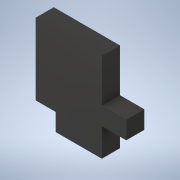
# Autodesk Inventor part: Remote Batery Spacer
Saved by Autodesk Inventor 2020 (Build 240168000, 168)
## iProperties
Created: 2019-06-21
Part Number: Remote Batery Spacer
Material: Generic
Document SubType Name: Modeling
Designer: LSabe
Density: 1 g/cm^3
Appearance: Default
Author: LSabe
Autodesk Inventor part; units mm, degrees
ref_plane "YZ Plane" through (0, 0, 0) normal (1, 0, 0) x (0, 1, 0)
ref_plane "XZ Plane" through (0, 0, 0) normal (0, 1, 0) x (-1, 0, 0)
sketch "Sketch1" plane through (0, 0, 0) normal (0, 0, 1) x (1, 0, 0)
  line L0 (11.176, -4.445) -> (1.27, -4.445)
  line L1 (-5.4348, 0) -> (-5.4348, -19.4068)
  line L2 (12.446, 0) -> (12.446, -11.684)
  line L3 (19.05, -11.684) -> (19.05, -16.51)
  line L4 (19.05, -16.51) -> (12.446, -16.51)
  line L5 (-4.1648, -1.27) -> (0, -1.27)
  line L6 (-4.1648, -18.1368) -> (-4.1648, -1.27)
  line L7 (0, -4.445) -> (0, -1.27)
  line L8 (1.27, -5.715) -> (11.176, -5.715)
  line L9 (11.176, -22.86) -> (1.27, -22.86)
  line L10 (1.27, -18.1368) -> (11.176, -18.1368)
  line L11 (12.446, -15.24) -> (17.78, -15.24)
  line L12 (17.78, -15.24) -> (17.78, -12.954)
  line L13 (17.78, -12.954) -> (12.446, -12.954)
  line L14 (11.176, -5.715) -> (11.176, -18.1368)
  line L15 (12.446, -15.24) -> (12.446, -12.954)
  line L16 (12.446, -15.24) -> (13.462, -15.24) construction
  line L17 (11.176, -4.445) -> (11.176, -1.27)
  line L18 (1.27, -4.445) -> (1.27, -1.27)
  line L19 (0, -18.1368) -> (0, -1.27)
  line L20 (1.27, -1.27) -> (11.176, -1.27)
  line L21 (1.27, -18.1368) -> (1.27, -5.715)
  line L22 (11.176, -22.86) -> (11.176, -19.4068)
  line L23 (1.27, -22.86) -> (1.27, -19.4068)
  line L24 (1.27, -22.86) -> (3.1836, -22.86) construction
  line L25 (12.446, 0) -> (-5.4348, 0)
  line L26 (12.446, -16.51) -> (12.446, -24.13)
  line L27 (0, -18.1368) -> (-4.1648, -18.1368)
  line L28 (12.446, -11.684) -> (19.05, -11.684)
  line L29 (12.446, -24.13) -> (0, -24.13)
  line L30 (0, -24.13) -> (0, -19.4068)
  line L31 (0, -19.4068) -> (-5.4348, -19.4068)
  line L32 (1.27, -19.4068) -> (11.176, -19.4068)
  point P0 (0, 0)
  point P1 (0, -10.414)
  point P2 (-4.1648, -10.414)
  constraints: 66 end point, 7 horizontal, 3 perpendicular, 3 vertical, 2 point on line, 1 parallel
extrude "Extrusion1" add sketch "Sketch1" along normal blind 3.8354
sketch "Sketch3" plane through (0, 0, 3.8354) normal (0, 0, 1) x (1, 0, 0)
  line L0 (19.05, -16.51) -> (19.05, -11.684)
  line L1 (19.05, -11.684) -> (12.446, -11.684)
  line L2 (12.446, -11.684) -> (12.446, 0)
  line L3 (12.446, 0) -> (-5.4348, 0)
  line L4 (-5.4348, 0) -> (-5.4348, -19.4068)
  line L5 (-5.4348, -19.4068) -> (0, -19.4068)
  line L6 (0, -19.4068) -> (0, -24.13)
  line L7 (0, -24.13) -> (12.446, -24.13)
  line L8 (12.446, -24.13) -> (12.446, -16.51)
  line L9 (12.446, -16.51) -> (19.05, -16.51)
  constraints: 20 end point
extrude "Extrusion3" add sketch "Sketch3" along normal blind 1.016
ref_plane "Work Plane1" through (6.223, -18.1368, 0) normal (-1, 0, 0) x (0, 0, 1)
body "Solid1"
